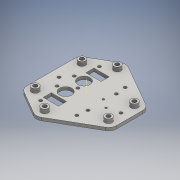
# Autodesk Inventor part: efector
Saved by Autodesk Inventor 2016 SP1 (Build 200210100, 210)
## iProperties
Created: 2016-03-06
Part Number: efector
Material: Generic
Document SubType Name: Modeling
Designer: roduino
Density: 1 g/cm^3
Appearance: Default
Author: roduino
Autodesk Inventor part; units mm, degrees
ref_plane "YZ Plane" through (0, 0, 0) normal (1, 0, 0) x (0, 1, 0)
ref_plane "XZ Plane" through (0, 0, 0) normal (0, 1, 0) x (-1, 0, 0)
ref_plane "XY Plane" through (0, 0, 0) normal (0, 0, 1) x (1, 0, 0)
sketch "Sketch1" plane through (0, 0, 0) normal (0, 0, 1) x (1, 0, 0)
  circle A0 centre (-12, 9) radius 6
  circle A1 centre (-12, -9) radius 6
  circle A2 centre (-28, 23) radius 2
  circle A3 centre (-28, -23) radius 2
  arc A4 (-31.4115, -18.0643) -> (-23.8208, -27.3051) centre (-28, -23) ccw
  arc A5 (-23.8208, 27.3051) -> (-31.4115, 18.0643) centre (-28, 23) ccw
  line L0 (-28, 23) -> (-28, -23) construction
  circle A6 centre (0, 0) radius 36.2353 construction
  arc A7 (-11.7365, -34.282) -> (0.0617, -36.2353) centre (-5.9186, -35.7487) ccw
  circle A8 centre (-5.9186, -35.7487) radius 2
  arc A9 (31.3499, -18.171) -> (35.5573, -6.9768) centre (33.9186, -12.7487) ccw
  circle A10 centre (33.9186, -12.7487) radius 2
  arc A11 (35.5573, 6.9768) -> (31.3499, 18.171) centre (33.9186, 12.7487) ccw
  circle A12 centre (33.9186, 12.7487) radius 2
  arc A13 (0.0617, 36.2353) -> (-11.7365, 34.282) centre (-5.9186, 35.7487) ccw
  circle A14 centre (-5.9186, 35.7487) radius 2
  line L1 (33.9186, 12.7487) -> (33.9186, -12.7487) construction
  line L2 (-34, 23) -> (-34, -23)
  line L3 (39.9186, 12.7487) -> (39.9186, -12.7487)
  line L4 (-31, 28.1962) -> (-8.9186, 40.9449)
  line L5 (-2.9186, 40.9449) -> (36.9186, 17.9449)
  line L6 (36.9186, -17.9449) -> (-2.9186, -40.9449)
  line L7 (-31, -28.1962) -> (-8.9186, -40.9449)
  dimension "d0" = 12
  dimension "d1" = 12
  dimension "d4" = 4
  dimension "d5" = 4
  dimension "d6" = 46
  dimension "d7" = 23
  dimension "d8" = 28
  dimension "d9" = 28
  dimension "d10" = 12
  dimension "d11" = 12
  dimension "d15" = 360
  dimension "d42" = 25.4974
  dimension "d45" = 9
  dimension "d46" = 9
  dimension "d48" = 22
  dimension "d49" = 22
  constraints: 29 point on circle, 16 end point, 15 centre point, 8 tangent, 7 coincident, 3 parallel, 1 vertical, 37 other
  measures "d0" diameter of A0
  measures "d1" diameter of A1
  measures "d4" diameter of A2
  measures "d5" diameter of A3
  measures "d6" distance of A3.centre A2.centre
  measures "d7" vertical distance of point (0, 0) A3.centre
  measures "d8" horizontal distance of point (0, 0) A2.centre
  measures "d9" horizontal distance of point (0, 0) A3.centre
  measures "d10" diameter of A4
  measures "d11" diameter of A5
  measures "d42" distance of A9.centre A11.centre
  measures "d45" vertical distance of point (0, 0) A0.centre
  measures "d46" vertical distance of point (0, 0) A1.centre
  measures "d48" distance from line of A0.centre L2
  measures "d49" distance from line of A1.centre L2
extrude "Extrusion1" add sketch "Sketch1" along normal blind 5
sketch "Sketch2" plane through (0, 0, 5) normal (0, 0, 1) x (1, 0, 0)
  circle A0 centre (-12, 9) radius 6 projected
  circle A1 centre (-12, -9) radius 6 projected
  circle A2 centre (-9, 0) radius 1.5
  circle A3 centre (-21, 8.5) radius 1.5
  circle A4 centre (-21, -8.5) radius 1.5
  point P0 (0, 0)
  dimension "d19" = 3
  dimension "d20" = 3
  dimension "d21" = 3
  dimension "d23" = 21
  dimension "d24" = 21
  dimension "d25" = 17
  dimension "d26" = 8.5
  dimension "d47" = 9
  constraints: 3 centre point
  measures "d19" diameter of A2
  measures "d20" diameter of A3
  measures "d21" diameter of A4
  measures "d23" horizontal distance of point (0, 0) A3.centre
  measures "d24" horizontal distance of point (0, 0) A4.centre
  measures "d25" distance of A4.centre A3.centre
  measures "d26" vertical distance of point (0, 0) A3.centre
  measures "d47" distance of point (0, 0) A2.centre
extrude "Extrusion2" cut sketch "Sketch2" against normal through all contours A2 | A3 | A4
sketch "Sketch3" plane through (0, 0, 5) normal (0, 0, 1) x (1, 0, 0)
  circle A0 centre (14.9186, 14) radius 1.5
  circle A1 centre (14.9186, -14) radius 1.5
  line L0 (39.9186, -12.7487) -> (39.9186, 12.7487) projected
  point P0 (0, 0)
  dimension "d29" = 3
  dimension "d30" = 3
  dimension "d31" = 28
  dimension "d33" = 14
  dimension "d77" = 25
  dimension "d78" = 25
  constraints: 2 centre point
  measures "d29" diameter of A0
  measures "d30" diameter of A1
  measures "d31" distance of A1.centre A0.centre
  measures "d33" vertical distance of point (0, 0) A1.centre
  measures "d77" distance from line of L0 A0.centre
  measures "d78" distance from line of L0 A1.centre
extrude "Extrusion3" cut sketch "Sketch3" against normal through all
sketch "Sketch6" plane through (0, 0, 5) normal (0, 0, 1) x (1, 0, 0)
  arc A0 (22.75, -18) -> (24.75, -16) centre (22.75, -16) ccw projected
  line L0 (22.75, -18) -> (17.25, -18) projected
  arc A1 (15.25, -16) -> (17.25, -18) centre (17.25, -16) ccw projected
  line L1 (15.25, -16) -> (15.25, 16) projected
  arc A2 (17.25, 18) -> (15.25, 16) centre (17.25, 16) ccw projected
  line L2 (17.25, 18) -> (22.75, 18) projected
  arc A3 (24.75, 16) -> (22.75, 18) centre (22.75, 16) ccw projected
  line L3 (24.75, 16) -> (24.75, -16) projected
  circle A4 centre (20, -14) radius 1.5 projected
  circle A5 centre (20, 14) radius 1.5 projected
  circle A6 centre (21.75, -3) radius 1 projected
  point P0 (0, 0)
extrude "Extrusion5" cut sketch "Sketch6" against normal through all contours A6
thread "Thread1" size "M4x0.7" class "6H" standard "ANSI Metric M Profile" full length
thread "Thread2" size "M4x0.7" class "6H" standard "ANSI Metric M Profile" full length
thread "Thread3" size "M4x0.7" class "6H" standard "ANSI Metric M Profile" full length
thread "Thread4" size "M4x0.7" class "6H" standard "ANSI Metric M Profile" full length
thread "Thread5" size "M4x0.7" class "6H" standard "ANSI Metric M Profile" full length
thread "Thread6" size "M4x0.7" class "6H" standard "ANSI Metric M Profile" full length
sketch "Sketch8" plane through (0, 0, 5) normal (0, 0, 1) x (1, 0, 0)
  circle A0 centre (-28, 23) radius 2 projected
  circle A1 centre (-5.9186, 35.7487) radius 2 projected
  circle A2 centre (33.9186, 12.7487) radius 2 projected
  circle A3 centre (33.9186, -12.7487) radius 2 projected
  circle A4 centre (-5.9186, -35.7487) radius 2 projected
  circle A5 centre (-28, -23) radius 2 projected
  circle A6 centre (21.75, -3) radius 1 projected
  circle A7 centre (14.9186, 14) radius 1.5 projected
  circle A8 centre (14.9186, -14) radius 1.5 projected
  circle A9 centre (-21, 8.5) radius 1.5 projected
  circle A10 centre (-9, 0) radius 1.5 projected
  circle A11 centre (-21, -8.5) radius 1.5 projected
  circle A12 centre (-12, -9) radius 6 projected
  circle A13 centre (-12, 9) radius 6 projected
  circle A14 centre (-5.9186, 35.7487) radius 2 projected
  circle A15 centre (33.9186, 12.7487) radius 2 projected
  circle A16 centre (33.9186, -12.7487) radius 2 projected
  circle A17 centre (-5.9186, -35.7487) radius 2 projected
  circle A18 centre (-28, -23) radius 2 projected
  circle A19 centre (-28, 23) radius 2 projected
  arc A20 (-31, 28.1962) -> (-34, 23) centre (-28, 23) ccw projected
  line L0 (-34, 23) -> (-34, -23) projected
  arc A21 (-34, -23) -> (-31, -28.1962) centre (-28, -23) ccw projected
  line L1 (-31, -28.1962) -> (-8.9186, -40.9449) projected
  arc A22 (-8.9186, -40.9449) -> (-2.9186, -40.9449) centre (-5.9186, -35.7487) ccw projected
  line L2 (-2.9186, -40.9449) -> (36.9186, -17.9449) projected
  arc A23 (36.9186, -17.9449) -> (39.9186, -12.7487) centre (33.9186, -12.7487) ccw projected
  line L3 (39.9186, -12.7487) -> (39.9186, 12.7487) projected
  arc A24 (39.9186, 12.7487) -> (36.9186, 17.9449) centre (33.9186, 12.7487) ccw projected
  line L4 (36.9186, 17.9449) -> (-2.9186, 40.9449) projected
  arc A25 (-2.9186, 40.9449) -> (-8.9186, 40.9449) centre (-5.9186, 35.7487) ccw projected
  line L5 (-8.9186, 40.9449) -> (-31, 28.1962) projected
  circle A26 centre (-28, 23) radius 3.5
  circle A27 centre (-5.9186, 35.7487) radius 3.5
  circle A28 centre (33.9186, 12.7487) radius 3.5
  circle A29 centre (33.9186, -12.7487) radius 3.5
  circle A30 centre (-5.9186, -35.7487) radius 3.5
  circle A31 centre (-28, -23) radius 3.5
  point P0 (0, 0)
  dimension "d62" = 1.5
  dimension "d63" = 1.5
  dimension "d64" = 1.5
  dimension "d65" = 1.5
  dimension "d66" = 1.5
  dimension "d67" = 1.5
  constraints: 6 centre point
  measures "d62" radial gap between concentric circles of A0 A26
  measures "d63" radial gap between concentric circles of A1 A27
  measures "d64" radial gap between concentric circles of A2 A28
  measures "d65" radial gap between concentric circles of A3 A29
  measures "d66" radial gap between concentric circles of A4 A30
  measures "d67" radial gap between concentric circles of A5 A31
extrude "Extrusion6" cut sketch "Sketch8" against normal blind 2 contours L5 A25 L4 A24 L3 A23 L2 A22 L1 A21 L0 A20
sketch "Sketch9" plane through (-28, -23, 5) normal (0, 0, 1) x (1, 0, 0)
  circle A0 centre (0, 0) radius 3.5 projected
  circle A1 centre (0, 46) radius 3.5 projected
  circle A2 centre (22.0814, 58.7487) radius 2 projected
  circle A3 centre (22.0814, 58.7487) radius 3.5 projected
  circle A4 centre (0, 46) radius 2 projected
  circle A5 centre (0, 0) radius 2 projected
  circle A6 centre (22.0814, -12.7487) radius 3.5 projected
  circle A7 centre (22.0814, -12.7487) radius 2 projected
  circle A8 centre (61.9186, 10.2513) radius 3.5 projected
  circle A9 centre (61.9186, 10.2513) radius 2 projected
  circle A10 centre (61.9186, 35.7487) radius 2 projected
  circle A11 centre (61.9186, 35.7487) radius 3.5 projected
  point P0 (28, 23)
extrude "Extrusion7" add sketch "Sketch9" along normal blind 2
sketch "Sketch10" plane through (0, 0, 3) normal (0, 0, 1) x (1, 0, 0)
  circle A0 centre (-12, 9) radius 6 projected
  circle A1 centre (-12, -9) radius 6 projected
  circle A2 centre (-28, -23) radius 3.5 projected
  circle A3 centre (-5.9186, -35.7487) radius 3.5 projected
  circle A4 centre (33.9186, -12.7487) radius 3.5 projected
  circle A5 centre (33.9186, 12.7487) radius 3.5 projected
  circle A6 centre (-5.9186, 35.7487) radius 3.5 projected
  circle A7 centre (-28, 23) radius 3.5 projected
  circle A8 centre (-21, -8.5) radius 1.5 projected
  circle A9 centre (-9, 0) radius 1.5 projected
  circle A10 centre (-21, 8.5) radius 1.5 projected
  circle A11 centre (14.9186, -14) radius 1.5 projected
  circle A12 centre (14.9186, 14) radius 1.5 projected
  circle A13 centre (21.75, -3) radius 1 projected
  arc A14 (-31, 28.1962) -> (-34, 23) centre (-28, 23) ccw projected
  line L0 (-34, -23) -> (-34, 23) projected
  arc A15 (-34, -23) -> (-31, -28.1962) centre (-28, -23) ccw projected
  line L1 (-8.9186, -40.9449) -> (-31, -28.1962) projected
  arc A16 (-8.9186, -40.9449) -> (-2.9186, -40.9449) centre (-5.9186, -35.7487) ccw projected
  line L2 (36.9186, -17.9449) -> (-2.9186, -40.9449) projected
  arc A17 (36.9186, -17.9449) -> (39.9186, -12.7487) centre (33.9186, -12.7487) ccw projected
  line L3 (39.9186, 12.7487) -> (39.9186, -12.7487) projected
  arc A18 (39.9186, 12.7487) -> (36.9186, 17.9449) centre (33.9186, 12.7487) ccw projected
  line L4 (-2.9186, 40.9449) -> (36.9186, 17.9449) projected
  arc A19 (-2.9186, 40.9449) -> (-8.9186, 40.9449) centre (-5.9186, 35.7487) ccw projected
  line L5 (-31, 28.1962) -> (-8.9186, 40.9449) projected
  arc A20 (-32, 29.9282) -> (-36, 23) centre (-28, 23) ccw
  line L6 (-32, 29.9282) -> (-9.9186, 42.6769)
  arc A21 (-1.9186, 42.6769) -> (-9.9186, 42.6769) centre (-5.9186, 35.7487) ccw
  line L7 (-1.9186, 42.6769) -> (37.9186, 19.6769)
  arc A22 (41.9186, 12.7487) -> (37.9186, 19.6769) centre (33.9186, 12.7487) ccw
  line L8 (41.9186, 12.7487) -> (41.9186, -12.7487)
  arc A23 (37.9186, -19.6769) -> (41.9186, -12.7487) centre (33.9186, -12.7487) ccw
  line L9 (37.9186, -19.6769) -> (-1.9186, -42.6769)
  arc A24 (-9.9186, -42.6769) -> (-1.9186, -42.6769) centre (-5.9186, -35.7487) ccw
  line L10 (-9.9186, -42.6769) -> (-32, -29.9282)
  arc A25 (-36, -23) -> (-32, -29.9282) centre (-28, -23) ccw
  line L11 (-36, -23) -> (-36, 23)
  point P0 (0, 0)
  dimension "d72" = 2
  constraints: 12 end point, 12 point on circle, 6 centre point, 11 other
  measures "d72" distance between parallel lines of L0 L11
extrude "Extrusion8" add sketch "Sketch10" against normal up to surface (3 mm away) contours L6 A21 L7 A22 L8 A23 L9 A24 L10 A25 L11 A20
sketch "Sketch11" plane through (0, 0, 0) normal (0, 0, -1) x (-1, 0, 0)
  circle A0 centre (-33.4186, 0) radius 1.5
  line L0 (-41.9186, 12.7487) -> (-41.9186, -12.7487) projected
  line L1 (0, 0) -> (-49.8844, 0) construction
  circle A1 centre (16.7093, -28.9413) radius 1.5
  circle A2 centre (16.7093, 28.9413) radius 1.5
  dimension "d97" = 8.5
  dimension "d98" = 0
  dimension "d101" = 360
  constraints: 3 centre point, 2 end point, 1 horizontal, 7 other
  measures "d97" distance from line of L0 A0.centre
  measures "d98" distance from line of L1 A0.centre
extrude "Extrusion9" cut sketch "Sketch11" against normal through all
sketch "Sketch12" plane through (0, 0, 3) normal (0, 0, 1) x (1, 0, 0)
  arc A0 (12.7181, 3.8928) -> (13.6045, 2.1) centre (13.1686, 3) ccw
  circle A1 centre (13.1686, 3) radius 1
  point P0 (0, 0)
  constraints: 2 centre point, 2 point on circle, 1 coincident, 1 concentric, 4 other
extrude "Extrusion10" cut sketch "Sketch12" against normal through all
sketch "Sketch13" plane through (0, 0, 0) normal (0, 0, -1) x (-1, 0, 0)
  line L0 (6, 15) -> (6, -15)
  line L1 (24, 15) -> (6, 15)
  line L2 (24, -15) -> (6, -15)
  line L3 (9.9186, -42.6769) -> (32, -29.9282) projected
  line L4 (3.1479, -25) -> (18.1479, -25)
  line L5 (18.1479, -25) -> (18.1479, -17)
  line L6 (18.1479, -17) -> (3.1479, -17)
  line L7 (3.1479, -17) -> (3.1479, -25)
  point P0 (0, 0)
  dimension "d84" = 8
  dimension "d85" = 15
  dimension "d86" = 2
  constraints: 14 end point, 3 horizontal, 2 parallel, 1 perpendicular, 1 vertical, 4 other
  measures "d84" distance of L6.end L4.start
  measures "d85" distance of L4.start L4.end
  measures "d86" distance between parallel lines of L2 L6
extrude "Extrusion11" cut sketch "Sketch13" against normal through all
mirror "Mirror1" about plane through (0, 0, 0) normal (0, 1, 0) of "Extrusion11"
sketch "Sketch14" plane through (0, 0, 3) normal (0, 0, 1) x (1, 0, 0)
  circle A0 centre (-27.5, 0) radius 1.5
  line L0 (-36, -23) -> (-36, 23) projected
  circle A1 centre (13.75, -23.8157) radius 1.5
  circle A2 centre (13.75, 23.8157) radius 1.5
  point P0 (0, 0)
  dimension "d89" = 3
  dimension "d90" = 8.5
  dimension "d93" = 360
  constraints: 3 centre point, 7 other
  measures "d89" diameter of A0
  measures "d90" distance from line of A0.centre L0
extrude "Extrusion12" cut sketch "Sketch14" against normal through all
equation "\"d1\" = d0"
equation "\"d5\" = d4"
equation "\"d7\" = 0.5 * d6"
equation "\"d9\" = d8"
equation "\"d10\" = d11"
equation "\"d46\" = d45"
equation "\"d49\" = d48"
equation "\"d24\" = d23"
equation "\"d26\" = 0.5 * d25"
equation "\"d33\" = 0.5 * d31"
equation "\"d78\" = d77"
body "Solid1"
